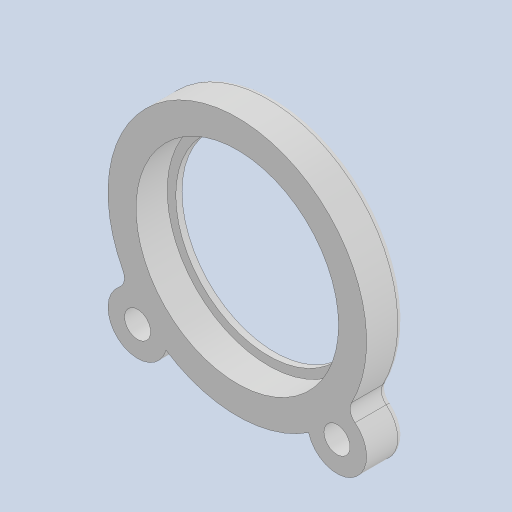
# Autodesk Inventor part: cage_inside_06
Saved by Autodesk Inventor 2024.4 (Build 284460030, 460C)
## iProperties
Created: 2026-07-27
Part Number: cage_inside_06
Material: Generic
Document SubType Name: Modeling
Designer: tooles01
Density: 1 g/cm^3
Appearance: Default
Author: tooles01
Autodesk Inventor part; units mm, degrees
ref_plane "YZ Plane" through (0, 0, 0) normal (1, 0, 0) x (0, 1, 0)
ref_plane "XZ Plane" through (0, 0, 0) normal (0, 1, 0) x (-1, 0, 0)
sketch "Sketch1: base" plane through (0, 0, 0) normal (0, 0, 1) x (1, 0, 0)
  circle A0 centre (-5, 4) radius 16.25
  circle A1 centre (-5, 4) radius 20.75
  circle A2 centre (-21, -12) radius 4.75
  circle A3 centre (11, -12) radius 4.75
  line L0 (-21, -12) -> (11, -12) construction
  line L1 (-21, 20) -> (-21, -12) construction
  point P0 (0, 0)
  point P1 (-5, -12)
  point P2 (-21, 4)
  point P3 (-22.3145, -7.4355)
  point P4 (-16.4355, -13.3145)
  point P5 (6.4355, -13.3145)
  point P6 (12.3145, -7.4355)
  dimension "d0" = 9.5
  dimension "d1" = 32
  dimension "d2" = 41.5
  dimension "d3" = 32.5
  dimension "d4" = 32
  constraints: 4 centre point, 4 end point, 3 coincident, 2 midpoint, 1 equal radius, 1 horizontal, 1 horizontal alignment, 1 perpendicular, 1 vertical alignment, 1 other
  measures "d0" diameter of A2
  measures "d1" distance of L0.start L0.end
  measures "d2" diameter of A1
  measures "d3" diameter of A0
  measures "d4" distance of L1.start L0.start
sketch "Sketch2: tube stopper" plane through (0, 0, 0) normal (0, 0, 1) x (1, 0, 0)
  circle A0 centre (-5, 4) radius 14.875
  circle A1 centre (-5, 4) radius 16.25 projected
  point P0 (0, 0)
  dimension "d14" = 29.75
  constraints: 1 centre point, 1 coincident
  measures "d14" diameter of A0
extrude "Ex1: base" add sketch "Sketch1: base" along normal blind 6
ref_plane "Work Plane1" through (0, 0, 0) normal (0, 0, 1) x (1, 0, 0)
sketch "Sketch: text" plane through (0, 0, 0) normal (0, 0, -1) x (-1, 0, 0)
  line L0 (3.25, 24) -> (6.75, 24) construction
  line L1 (6.75, 24) -> (6.75, 20.5) construction
  line L2 (6.75, 20.5) -> (3.25, 20.5) construction
  line L3 (3.25, 20.5) -> (3.25, 24) construction
  line L4 (2.1748, 22.9624) -> (3.0901, 22.9624)
  line L5 (3.0901, 22.9624) -> (3.5386, 21.5071)
  line L6 (3.5386, 21.5071) -> (3.9993, 22.9624)
  line L7 (3.9993, 22.9624) -> (4.8871, 22.9624)
  line L8 (4.8871, 22.9624) -> (3.9108, 20.665)
  line L9 (3.9108, 20.665) -> (3.1297, 20.665)
  line L10 (3.1297, 20.665) -> (2.1748, 22.9624)
  line L11 (7.6056, 23.1211) -> (6.7299, 23.0143)
  spline S0 degree 2 poles (6.7299, 23.0143) (6.6964, 23.1973) (6.5347, 23.3499) (6.4157, 23.3499) knots 0 0 0 1 2 2 2
  spline S1 degree 2 poles (6.4157, 23.3499) (6.2021, 23.3499) (6.0831, 23.1333) knots 0 0 0 1 1 1
  spline S2 degree 2 poles (6.0831, 23.1333) (5.9946, 22.9777) (5.955, 22.4651) knots 0 0 0 1 1 1
  spline S3 degree 2 poles (5.955, 22.4651) (6.1136, 22.6268) (6.4462, 22.7794) (6.6628, 22.7794) knots 0 0 0 1 2 2 2
  spline S4 degree 2 poles (6.6628, 22.7794) (7.0869, 22.7794) (7.6727, 22.1753) (7.6727, 21.7084) knots 0 0 0 1 2 2 2
  spline S5 degree 2 poles (7.6727, 21.7084) (7.6727, 21.3942) (7.3767, 20.8755) (6.852, 20.6101) (6.4553, 20.6101) knots 0 0 0 1 2 3 3 3
  spline S6 degree 2 poles (6.4553, 20.6101) (5.9794, 20.6101) (5.4058, 20.9335) (5.061, 21.6474) (5.061, 22.2332) knots 0 0 0 1 2 3 3 3
  spline S7 degree 2 poles (5.061, 22.2332) (5.061, 23.0906) (5.7841, 23.8899) (6.4218, 23.8899) knots 0 0 0 1 2 2 2
  spline S8 degree 2 poles (6.4218, 23.8899) (6.8001, 23.8899) (7.2394, 23.716) (7.5293, 23.3773) (7.6056, 23.1211) knots 0 0 0 1 2 3 3 3
  spline S9 degree 2 poles (5.9855, 21.7084) (5.9855, 21.4522) (6.2448, 21.1593) (6.4309, 21.1593) knots 0 0 0 1 2 2 2
  spline S10 degree 2 poles (6.4309, 21.1593) (6.6048, 21.1593) (6.8367, 21.4217) (6.8367, 21.684) knots 0 0 0 1 2 2 2
  spline S11 degree 2 poles (6.8367, 21.684) (6.8367, 21.9525) (6.5957, 22.2332) (6.4157, 22.2332) knots 0 0 0 1 2 2 2
  spline S12 degree 2 poles (6.4157, 22.2332) (6.2326, 22.2332) (5.9855, 21.9617) (5.9855, 21.7084) knots 0 0 0 1 2 2 2
  point P0 (0, 0)
  point P1 (5, 4)
  point P2 (5, 20.5)
  dimension "d22" = 3.5
  dimension "d23" = 16.5
  constraints: 1 midpoint, 1 perpendicular, 1 vertical, 1 vertical alignment, 2 other
  measures "d22" distance of L0.start L0.end
  measures "d23" distance from line of point (5, 4) L2
hole "Hole1: M3 heat-sets" at (11, -12, 0) at (-21, -12, 0) direction (0, 0, -1) diameter 4.2 end through all both
extrude "Ex: tube stopper" add sketch "Sketch2: tube stopper" along normal blind 1
fillet "Fillet1" radius 2 2 edges at (12.3145, -7.4355, 3) (-22.3145, -7.4355, 3)
fillet "Fillet2" radius 1 5 edges at (-23.1529, -7.0697, 0) (-23.6764, -15.9242, 0) (13.1529, -7.0697, 0) (13.6764, -15.9242, 0) (-5, 24.75, 0)
extrude "Ex: text" cut sketch "Sketch: text" against normal blind 1
body "Solid1"
